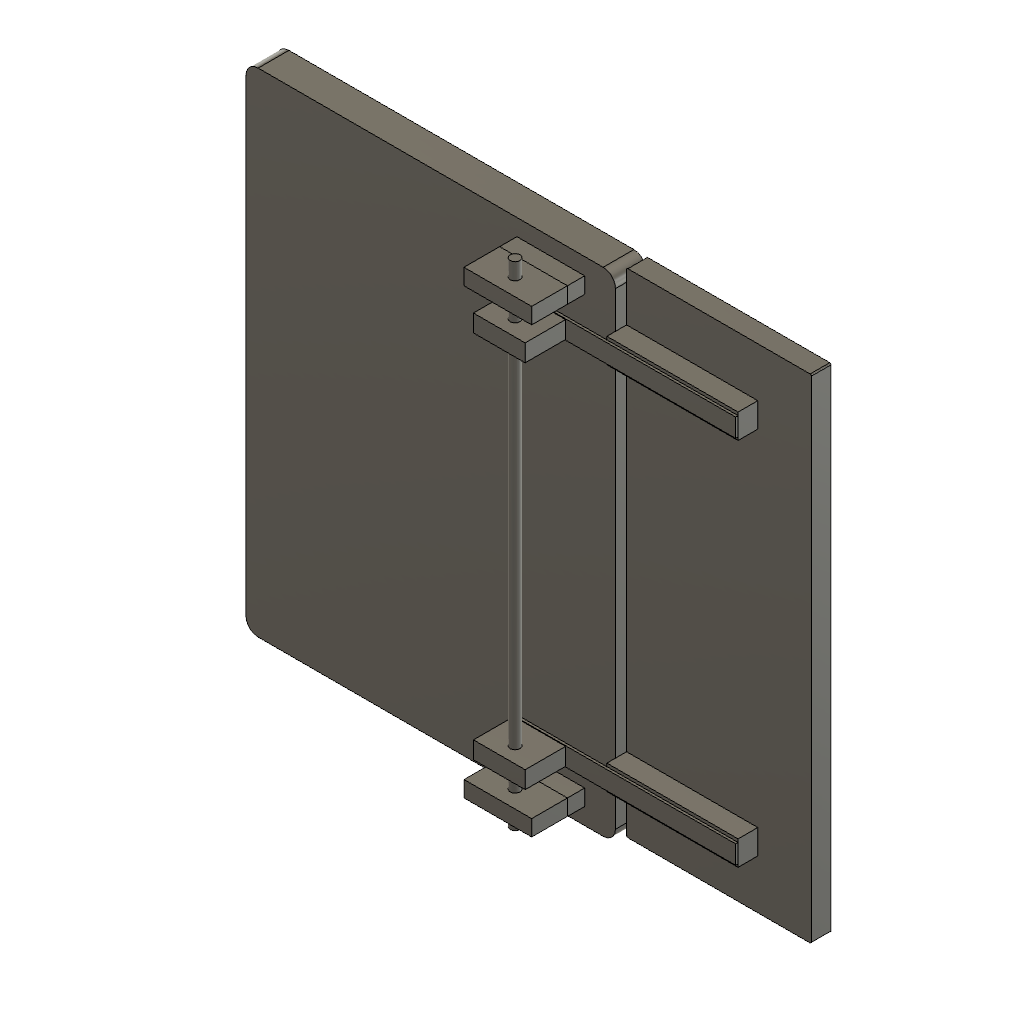
table_template (Autodesk Fusion 360 design; units mm, degrees)
part number: 2026-09-07-22-54-19-827
part number: 2026-09-07-22-54-19-966
part number: 2026-09-07-22-54-19-972
part number: 2026-09-07-22-54-20-006
part number: 2026-09-07-22-54-20-091
Autodesk Fusion 360 part; units mm, degrees
sketch "Sketch1" plane through (0, 0, 0) normal (0, 1, 0) x (1, 0, 0) in component "Base"
  line L0 (-247.5, 54) -> (52.5, 54)
  line L1 (52.5, 54) -> (52.5, 29)
  line L2 (52.5, 29) -> (-247.5, 29)
  line L3 (-247.5, 29) -> (-247.5, 54)
extrude "Extrude1" add sketch "Sketch1" along normal mid plane 400 makes body 1 in component "Base"
fillet "Fillet1" radius 10 4 edges at (-247.5, -200, -41.5) (52.5, -200, -41.5) (-247.5, 200, -41.5) (52.5, 200, -41.5) on bodies 1 in component "Base"
sketch "Sketch1 (2)" plane through (0, 0, 0) normal (0, 1, 0) x (1, 0, 0) in component "KP08"
  line L0 (-27.5, 15) -> (27.5, 15)
  line L1 (27.5, 15) -> (27.5, -14)
  line L2 (27.5, -14) -> (-27.5, -14)
  line L3 (-27.5, -14) -> (-27.5, 15)
  circle A0 centre (0, 0) radius 4
extrude "Extrude1'" add sketch "Sketch1 (2)" along normal mid plane 13 separate body makes body 2 in component "KP08"
sketch "Sketch2" plane through (0, 0, 0) normal (0, 1, 0) x (1, 0, 0) in component "KP08"
  line L0 (-27.5, 29) -> (27.5, 29)
  line L1 (27.5, 29) -> (27.5, 15)
  line L2 (27.5, 15) -> (-27.5, 15)
  line L3 (-27.5, 15) -> (-27.5, 29)
extrude "Extrude2" add sketch "Sketch2" along normal mid plane 13 separate body makes body 3 in component "KP08"
sketch "Sketch1 (3)" plane through (0, 0, 0) normal (0, 1, 0) x (1, 0, 0) in component "Swing"
  circle A0 centre (0, 0) radius 4
extrude "Extrude1''" add sketch "Sketch1 (3)" along normal mid plane 400 separate body makes body 4 in component "Swing"
sketch "Sketch2 (2)" plane through (0, 0, 0) normal (0, 1, 0) x (1, 0, 0) in component "Swing"
  line L0 (52.5, 54) -> (202.5, 54)
  line L1 (202.5, 54) -> (202.5, 38)
  line L2 (202.5, 38) -> (52.5, 38)
  line L3 (52.5, 38) -> (52.5, 54)
extrude "Extrude2'" add sketch "Sketch2 (2)" along normal mid plane 400 separate body makes body 5 in component "Swing"
fillet "Fillet1'" radius 1 4 edges at (52.5, -200, -46) (202.5, -200, -46) (52.5, 200, -46) (202.5, 200, -46) on bodies 5 in component "Swing"
sketch "Sketch1 (4)" plane through (0, 0, 0) normal (0, 1, 0) x (1, 0, 0) in component "SK8-hand-holder"
  line L0 (-21, 20) -> (21, 20)
  line L1 (21, 20) -> (21, -12.8)
  line L2 (21, -12.8) -> (-21, -12.8)
  line L3 (-21, -12.8) -> (-21, 20)
  circle A0 centre (0, 0) radius 4
extrude "Extrude1'''" add sketch "Sketch1 (4)" along normal mid plane 14 separate body makes body 6 in component "SK8-hand-holder"
sketch "Sketch2 (3)" plane through (0, 0, 0) normal (0, 1, 0) x (1, 0, 0) in component "SK8-hand-holder"
  line L0 (-21, 22) -> (159, 22)
  line L1 (159, 22) -> (159, 20)
  line L2 (159, 20) -> (-21, 20)
  line L3 (-21, 20) -> (-21, 22)
extrude "Extrude2''" add sketch "Sketch2 (3)" along normal mid plane 15 separate body makes body 7 in component "SK8-hand-holder"
sketch "Sketch3" plane through (0, 0, 0) normal (0, 1, 0) x (1, 0, 0) in component "SK8-hand-holder"
  line L0 (52.5, 38) -> (159, 38)
  line L1 (159, 38) -> (159, 22)
  line L2 (159, 22) -> (52.5, 22)
  line L3 (52.5, 22) -> (52.5, 38)
extrude "Extrude3" add sketch "Sketch3" along normal mid plane 20 separate body makes body 8 in component "SK8-hand-holder"
component "Base" placed x (1, 0, 0) y (0, 1, 0) z (0, 0, 1) at (0, 0, 0)
component "Swing" placed x (1, 0, 0) y (0, 1, 0) z (0, 0, 1) at (0, 0, 0)
component "KP08" placed x (1, 0, 0) y (0, 1, 0) z (0, 0, 1) at (0, 180, 0) in component "Base"
component "KP08" placed x (1, 0, 0) y (0, 1, 0) z (0, 0, 1) at (0, -180, 0) in component "Base"
component "SK8-hand-holder" placed x (1, 0, 0) y (0, 1, 0) z (0, 0, 1) at (0, 150, 0) in component "Swing"
component "SK8-hand-holder" placed x (1, 0, 0) y (0, 1, 0) z (0, 0, 1) at (0, -150, 0) in component "Swing"
named bodies: "Table", "kp08", "stand", "Shaft", "Panel", "sk8", "hand", "panelHolder"
